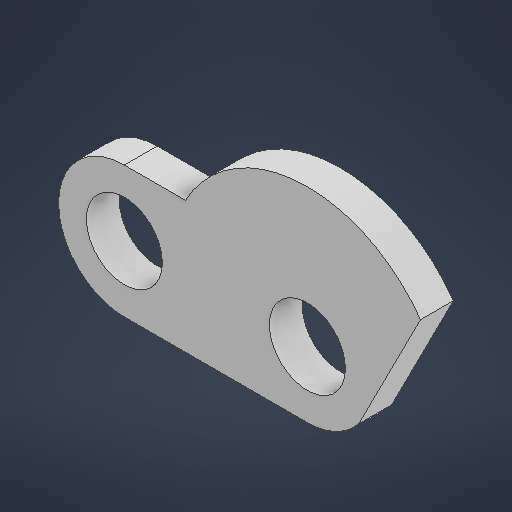
# Autodesk Inventor part: Arm Link Gear
Saved by Autodesk Inventor 2026.2 (Build 302298010, 298A)
## iProperties
Created: 2026-05-28
Part Number: Arm Link Gear
Material: Generic
Document SubType Name: Modeling
Designer: yassi
Density: 1 g/cm^3
Appearance: Default
Author: yassi
Autodesk Inventor part; units mm, degrees
ref_plane "YZ Plane" through (0, 0, 0) normal (1, 0, 0) x (0, 1, 0)
ref_plane "XZ Plane" through (0, 0, 0) normal (0, 1, 0) x (-1, 0, 0)
ref_plane "XY Plane" through (0, 0, 0) normal (0, 0, 1) x (1, 0, 0)
sketch "Sketch2" plane through (0, 0, 0) normal (0, 0, 1) x (1, 0, 0)
  circle A0 centre (0, 0) radius 5.2
  line L0 (0, 0) -> (25.045, 0)
  circle A1 centre (25.045, 0) radius 5.2
  circle A2 centre (0, 0) radius 9
  line L1 (0, 9) -> (8.364, 9)
  line L2 (0, -9) -> (25, -9)
  arc A3 (25, -9) -> (32.0761, -5.6183) centre (25.045, 0) ccw
  line L3 (32.0761, -5.6183) -> (50.6341, -5.6183) construction
  arc A4 (40.5237, 10.9392) -> (8.364, 9) centre (25.045, 0) ccw
  line L4 (32.0761, -5.6183) -> (40.5237, 10.9392)
  dimension "d0" = 10.4
  dimension "d1" = 25.045
  dimension "d2" = 10.4
  dimension "d3" = 18
  dimension "d4" = 8.364
  dimension "d5" = 25
  dimension "d12" = 18.588
  constraints: 10 end point, 6 point on circle, 5 centre point, 4 coincident, 4 horizontal, 1 tangent
  measures "d0" diameter of A0
  measures "d1" distance of L0.start L0.end
  measures "d2" diameter of A1
  measures "d3" diameter of A2
  measures "d4" distance of L1.start L1.end
  measures "d5" distance of L2.start L2.end
  measures "d12" distance of L4.end L3.start
extrude "Extrusion1" add sketch "Sketch2" along normal blind 4.5
derived "Assembly for Link Gear.iam"
body "Solid1"
